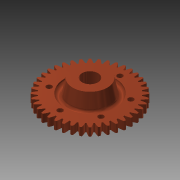
# Autodesk Inventor part: 平歯車11_
Saved by Autodesk Inventor 2013 (Build 170138000, 138)
## iProperties
Created: 2013-02-07
Part Number: 平歯車11_
Material: 銅、合金
Document SubType Name: Modeling
Designer: JohnHenry
Categories: <?xml version="1.0" encoding="UTF-16"?> <MemberInstance><Categories><FamilyTemplate><FamilyTemplateParameter ValueType="xs:double" Id="1" ObjectReferenceKey="da_z" ObjectType="kUserParameterObject"/><FamilyTemplateParameter ValueType="xs:double" Id="2" ObjectReferenceKey="da_b" ObjectType="kUserParameterObject"/><FamilyTemplateParameter ValueType="xs:double" Id="3" ObjectReferenceKey="da_beta" ObjectType="kUserParameterObject"/><FamilyTemplateParameter ValueType="xs:double" Id="4" ObjectReferenceKey="da_da" ObjectType="kUserParameterObject"/><FamilyTemplateParameter ValueType="xs:double" Id="5" ObjectReferenceKey="da_aw" ObjectType="kUserParameterObject"/><FamilyTemplateParameter ValueType="xs:string" Id="6" ObjectReferenceKey="EAIAABAAAACIAQAAAAAAAIAAAAAAAAAA" ObjectType="83910656" SubObjectId="SurfaceGeometry"/></FamilyTemplate><ParamToTemplateMap><ParamToTemplate CategoryParameter="//CategoryParameter[@InternalName='046C89C9-8512-4d59-83FE-43B91F4F132A']" TemplateParameter="1"/><ParamToTemplate CategoryParameter="//CategoryParameter[@InternalName='2552DF32-E462-4b46-AEBF-C6C7768E72AC']" TemplateParameter="2"/><ParamToTemplate CategoryParameter="//CategoryParameter[@InternalName='C9EE641D-15FC-4fae-A226-E94C4372FDD7']" TemplateParameter="3"/><ParamToTemplate><ParamToTemplate CategoryParameter="//CategoryParameter[@InternalName='00B6519A-459B-49c7-AD84-2E56D39A5744']" ConstantValue="0.063537"/></ParamToTemplate><ParamToTemplate><ParamToTemplate CategoryParameter="//CategoryParameter[@InternalName='04B31F0E-C7A6-4894-AA32-9629BEFACF47']" ConstantValue="1.000000"/></ParamToTemplate><ParamToTemplate><ParamToTemplate CategoryParameter="//CategoryParameter[@InternalName='43CBEC2E-7847-49e7-A936-2F7889FCB2D9']" ConstantValue="0.250000"/></ParamToTemplate><ParamToTemplate><ParamToTemplate CategoryParameter="//CategoryParameter[@InternalName='B1EFC894-105D-4ebd-86BF-FA20ED196853']" ConstantValue="0.350000"/></ParamToTemplate><ParamToTemplate><ParamToTemplate CategoryParameter="//CategoryParameter[@InternalName='51175063-3D10-4879-93E8-6246FE8B403D']" ConstantValue="2060000000.000000"/></ParamToTemplate><ParamToTemplate><ParamToTemplate CategoryParameter="//CategoryParameter[@InternalName='A3A52E27-4454-46a9-B0BD-C932399B70AF']" ConstantValue="0.300000"/></ParamToTemplate><ParamToTemplate><ParamToTemplate CategoryParameter="//CategoryParameter[@InternalName='91B76062-C214-41d9-B1B9-14D2AB99603D']" ConstantValue="0.075000"/></ParamToTemplate><ParamToTemplate><ParamToTemplate CategoryParameter="//CategoryParameter[@InternalName='374E806E-8B8A-4dda-A9AA-1039D6500AD2']" ConstantValue="13.333333"/></ParamToTemplate><ParamToTemplate><ParamToTemplate CategoryParameter="//CategoryParameter[@InternalName='2D373A89-B862-43d6-8D0B-0CBF12AB9F6C']" ConstantValue="0.349066"/></ParamToTemplate><ParamToTemplate CategoryParameter="//CategoryParameter[@InternalName='37777632-D6A2-4fac-9D53-DB8ACD95C989']" TemplateParameter="4"/><ParamToTemplate CategoryParameter="//CategoryParameter[@InternalName='FD1017F1-B727-4f7e-9707-0F86F1FF9423']" TemplateParameter="5"/><ParamToTemplate><ParamToTemplate CategoryParameter="//CategoryParameter[@InternalName='9E1B4470-B2D3-4ff1-B813-535BB4CDF51A']" ConstantValue="3520000.000000"/></ParamToTemplate><ParamToTemplate><ParamToTemplate CategoryParameter="//CategoryParameter[@InternalName='F8452263-BFF6-458c-9FB1-07C4B99E95CD']" ConstantValue="11400000.000000"/></ParamToTemplate><ParamToTemplate><ParamToTemplate CategoryParameter="//CategoryParameter[@InternalName='3E3BB259-FD49-497f-8171-6EBC954A3479']" ConstantValue="2.000000"/></ParamToTemplate><ParamToTemplate CategoryParameter="//CategoryParameter[@InternalName='27C3BAF2-7550-4e4b-AE2C-0DB134B7D9B7']" TemplateParameter="6"/></ParamToTemplateMap><Category DisplayName="Gear" InternalName="DC85795E-93AB-48d5-8EEE-5A27447B64BD" Mnemonic="Gear"><CategoryParameter DisplayName="z" InternalName="046C89C9-8512-4d59-83FE-43B91F4F132A" Mnemonic="z"/><CategoryParameter DisplayName="b" InternalName="2552DF32-E462-4b46-AEBF-C6C7768E72AC" Mnemonic="b"/><CategoryParameter DisplayName="||b|" InternalName="C9EE641D-15FC-4fae-A226-E94C4372FDD7" Mnemonic="beta"/><CategoryParameter DisplayName="x" InternalName="00B6519A-459B-49c7-AD84-2E56D39A5744" Mnemonic="x"/><CategoryParameter DisplayName="a*" InternalName="04B31F0E-C7A6-4894-AA32-9629BEFACF47" Mnemonic="a"/><CategoryParameter DisplayName="c*" InternalName="43CBEC2E-7847-49e7-A936-2F7889FCB2D9" Mnemonic="c"/><CategoryParameter DisplayName="r|.f|*" InternalName="B1EFC894-105D-4ebd-86BF-FA20ED196853" Mnemonic="rf"/><CategoryParameter DisplayName="E" InternalName="51175063-3D10-4879-93E8-6246FE8B403D" Mnemonic="E"/><CategoryParameter DisplayName="||m|" InternalName="A3A52E27-4454-46a9-B0BD-C932399B70AF" Mnemonic="mi"/><Category DisplayName="SpurGear" InternalName="26C5A22E-A91E-4dfd-A3B3-23CCAFAE1764" Mnemonic="SpurGear"><CategoryParameter DisplayName="m" InternalName="91B76062-C214-41d9-B1B9-14D2AB99603D" Mnemonic="m"/><CategoryParameter DisplayName="P" InternalName="374E806E-8B8A-4dda-A9AA-1039D6500AD2" Mnemonic="PP"/><CategoryParameter DisplayName="||a|" InternalName="2D373A89-B862-43d6-8D0B-0CBF12AB9F6C" Mnemonic="alpha"/><CategoryParameter DisplayName="d|.a|" InternalName="37777632-D6A2-4fac-9D53-DB8ACD95C989" Mnemonic="da"/><CategoryParameter DisplayName="a|.w|" InternalName="FD1017F1-B727-4f7e-9707-0F86F1FF9423" Mnemonic="aw"/><CategoryParameter DisplayName="||s||.Flim|" InternalName="9E1B4470-B2D3-4ff1-B813-535BB4CDF51A" Mnemonic="sFlim"/><CategoryParameter DisplayName="||s||.Hlim|" InternalName="F8452263-BFF6-458c-9FB1-07C4B99E95CD" Mnemonic="sHlim"/><CategoryParameter DisplayName="種類" InternalName="3E3BB259-FD49-497f-8171-6EBC954A3479" Mnemonic="type"/><CategoryParameter DisplayName="PitchDiameter" InternalName="27C3BAF2-7550-4e4b-AE2C-0DB134B7D9B7" Mnemonic="IDS_PITCHDIAM"/></Category></Category></Categories></MemberInstance>
Density: 7.15 g/cm^3
Mass: 17.9533 g
Surface Area: 24.2308 cm^2
Volume: 2.51094 cm^3
CustomPartVersion: 1
Author: JohnHenry
Autodesk Inventor part; units mm, degrees
sketch "Sketch1" plane through (0, 0, 0) normal (0, 0, 1) x (1, 0, 0)
  circle A0 centre (0, 0) radius 15.7977
  dimension "d0" = 31.5953
  constraints: 1 centre point
  measures "d0" diameter of A0
extrude "Extrusion1" add sketch "Sketch1" along normal blind 3
ref_plane "Work Plane2" through (0, 0, 1.5) normal (0, 0, 1) x (1, 0, 0)
sketch "Sketch2" plane through (0, 0, 0) normal (0, 0, -1) x (-1, 0, 0)
  circle A0 centre (0, 0) radius 15.7977 projected
  circle A1 centre (0, 0) radius 15
  dimension "d3" = 30
  constraints: 1 centre point, 1 coincident
  measures "d3" diameter of A1
surface extrude "ピッチ円直径" sketch "Sketch2" against normal through all shown no curves A1
ref_plane "Work Plane8" through (0, 0, 0) normal (0.9969173, 0.0784591, 0) x (0, 0, 1)
ref_plane "Work Plane9" through (0, 0, 0) normal (1, 0, 0) x (0, 1, 0)
spur gear teeth "平歯車" teeth 40 pitch diameter 30 tip diameter 31.5953 root diameter 28.2203 face width 3 start plane through (0, 0, 0) normal (0, 0, -1) x (-1, 0, 0)
sketch "スケッチ5" plane through (0, 0, 3) normal (0, 0, 1) x (1, 0, 0)
  arc A0 (-2.1645, 15.6487) -> (-2.7772, 15.5516) centre (0, 0) ccw projected
  constraints: 1 coincident
hole "Hole2" at (0, 0, 3) direction (0, 0, -1) diameter 6 end through all
sketch "スケッチ7" plane through (0, 0, 3) normal (0, 0, 1) x (1, 0, 0)
  arc A0 (-2.1645, 15.6487) -> (-2.7772, 15.5516) centre (0, 0) ccw projected
  circle A1 centre (0, 0) radius 11.25
  point P0 (0, 11.25)
  point P1 (-9.7428, 5.625)
  point P2 (-9.7428, -5.625)
  point P3 (0, -11.25)
  point P4 (9.7428, -5.625)
  point P5 (9.7428, 5.625)
  dimension "d77" = 22.5
  dimension "d80" = 360
  constraints: 1 coincident, 1 vertical alignment, 9 other
hole "Hole4" at (0, 11.25, 3) at (-9.7428, 5.625, 3) at (-9.7428, -5.625, 3) at (0, -11.25, 3) at (9.7428, -5.625, 3) at (9.7428, 5.625, 3) direction (0, 0, -1) diameter 2 depth 8 tip angle 118
sketch "スケッチ8" plane through (0, 0, 3) normal (0, 0, 1) x (1, 0, 0)
  arc A0 (1.383, 14.0422) -> (0.8307, 14.0857) centre (0, 0) ccw projected
  circle A1 centre (1.1071, 14.0667) radius 0.277
  dimension "d89" = 0.5541
  constraints: 1 centre point, 1 point on circle
  measures "d89" diameter of A1
extrude "押し出し3" cut sketch "スケッチ8" against normal through all
pattern_circular "放射状パターン1" count 40 over 360 about axis through (0, 0, -41.7831) along (0, 0, 1) of "押し出し3"
sketch "スケッチ12" plane through (0, 0, 3) normal (0, 0, 1) x (1, 0, 0)
  circle A0 centre (0, 0) radius 3 projected
  arc A1 (5.1758, 14.9257) -> (4.5858, 15.1174) centre (0, 0) ccw projected
  circle A2 centre (0, 0) radius 3
  circle A3 centre (0, 0) radius 7.5
  dimension "d109" = 15
  constraints: 2 centre point, 2 coincident, 1 concentric
  measures "d109" diameter of A3
extrude "押し出し7" add sketch "スケッチ12" along normal blind 5
chamfer "面取り2" distance 5 distance2 1 1 edges at (-7.5, 0, 8) measured on face at (7.4029, -1.2031, 6.3333)
sketch "スケッチ13" plane through (0, 0, 3) normal (0, 0, 1) x (1, 0, 0)
  circle A0 centre (0, 0) radius 7.5 projected
  arc A1 (5.1758, 14.9257) -> (4.5858, 15.1174) centre (0, 0) ccw projected
  circle A2 centre (0, 0) radius 9.5
  dimension "d115" = 19
  constraints: 1 centre point, 1 coincident
  measures "d115" diameter of A2
extrude "押し出し8" cut sketch "スケッチ13" against normal blind 1
fillet "フィレット1" radius 1 2 edges at (-7.5, 0, 2) (-9.5, 0, 2)
equation "\"d0\" = da_da"
equation "\"d1\" = da_b"
equation "\"d3\" = da_dw"
equation "\"da_da\" = 31.595305"
equation "\"da_b\" = 3"
equation "\"da_dw\" = 30"
body "Solid1"
body "Srf1"
